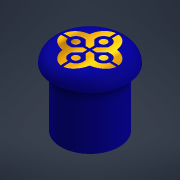
# Autodesk Inventor part: tutup
Saved by Autodesk Inventor 2021.3 (Build 253353000, 353)
## iProperties
Created: 2021-10-17
Part Number: tutup
Material: Rubber
Document SubType Name: Modeling
Designer: ASUS
Density: 0.93 g/cm^3
Appearance: Rubber - Black - Version 1.1
Author: ASUS
Autodesk Inventor part; units mm, degrees
ref_plane "YZ Plane" through (0, 0, 0) normal (1, 0, 0) x (0, 1, 0)
ref_plane "XY Plane" through (0, 0, 0) normal (0, 0, 1) x (1, 0, 0)
sketch "Sketch3" plane through (0, 0, 0) normal (0, 0, 1) x (1, 0, 0)
  line L0 (0, 0) -> (9.5, 0)
  line L1 (0, -15) -> (7.5, -15)
  line L2 (7.5, -15) -> (7.5, 0)
  line L3 (0, -15) -> (0, 3)
  line L4 (9.5, 0) -> (9.5, 0)
  line L5 (0, 3) -> (6.5, 3)
  line L6 (9.5, 0) -> (9.5, 0)
  arc A0 (9.5, 0) -> (6.5, 3) centre (6.5, 0) ccw
  dimension "d6" = 9.5
  dimension "d7" = 7.5
  dimension "d39" = 3
  dimension "d40" = 15
  dimension "d41" = 3
  constraints: 14 end point, 3 horizontal, 2 perpendicular, 2 point on circle, 2 tangent, 2 vertical, 1 centre point, 1 point on line
  measures "d6" distance of L0.start L0.end
  measures "d7" distance of L1.start L1.end
  measures "d39" distance of L0.start L3.end
  measures "d40" distance of L1.start L0.start
  measures "d41" radius of A0
revolve "Revolution1" add sketch "Sketch3" angle 360 about axis through (0, -15, 0) along (0, 1, 0)
ref_plane "Work Plane1" through (0, 5.5, 0) normal (0, 1, 0) x (-1, 0, 0)
sketch "Sketch4" plane through (0, 5.5, 0) normal (0, 1, 0) x (-1, 0, 0)
  line L0 (-9, -9) -> (9, -9) construction
  line L1 (9, -9) -> (9, 9) construction
  line L2 (9, 9) -> (-9, 9) construction
  line L3 (-9, 9) -> (-9, -9) construction
  point P0 (0, 0)
  dimension "d70" = 18
  dimension "d74" = 9
  dimension "d75" = 9
  constraints: 2 other
  measures "d70" distance of L0.end L0.start
  measures "d74" horizontal distance of L0.start point (0, 0)
  measures "d75" horizontal distance of L2.end point (0, 0)
decal "Decal3"
body "Solid2"
